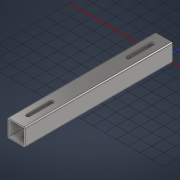
# Autodesk Inventor part: member_vertical
Saved by Autodesk Inventor 2021 (Build 250183000, 183)
## iProperties
Created: 2021-06-01
Part Number: member_vertical
Material: Steel, Galvanized
Document SubType Name: Modeling
Designer: Watchdog
Density: 7.85 g/cm^3
Appearance: Galvanized
Author: Watchdog
Autodesk Inventor part; units mm, degrees
ref_plane "YZ Plane" through (0, 0, 0) normal (1, 0, 0) x (0, 1, 0)
ref_plane "XZ Plane" through (0, 0, 0) normal (0, 1, 0) x (-1, 0, 0)
ref_plane "XY Plane" through (0, 0, 0) normal (0, 0, 1) x (1, 0, 0)
sketch "Sketch1" plane through (0, 0, 0) normal (0, 0, 1) x (1, 0, 0)
  line L0 (-15, 15) -> (15, 15)
  line L1 (15, 15) -> (15, -15)
  line L2 (15, -15) -> (-15, -15)
  line L3 (-15, -15) -> (-15, 15)
  line L4 (12.5, 12.5) -> (-12.5, 12.5)
  line L5 (-12.5, 12.5) -> (-12.5, -12.5)
  line L6 (-12.5, -12.5) -> (12.5, -12.5)
  line L7 (12.5, -12.5) -> (12.5, 12.5)
  point P0 (0, 0)
  dimension "d0" = 30
  dimension "d1" = 30
  dimension "d2" = 15
  dimension "d3" = 15
  dimension "d4" = 2.5
  constraints: 16 end point, 4 parallel, 2 perpendicular, 1 horizontal, 3 other
  measures "d0" distance of L0.start L0.end
  measures "d1" distance of L2.end L0.start
  measures "d2" distance from line of point (0, 0) L0
  measures "d3" distance from line of point (0, 0) L3
  measures "d4" distance between parallel lines of L0 L4
extrude "Extrusion1" add sketch "Sketch1" along normal blind 1000
fillet "Fillet1" radius 2 4 edges at (15, 15, 500) (-15, 15, 500) (-15, -15, 500) (15, -15, 500)
ref_plane "Work Plane1" through (0, 0, 250) normal (0, 0, -1) x (-1, 0, 0)
split "Split1" plane through (0, 0, 250) removes the side toward (0, 0, 1)
ref_plane "midPlane" through (-13, -15, 125) normal (0, 0, 1) x (1, 0, 0)
sketch "Sketch3" plane through (-13, 15, 0) normal (0, 1, 0) x (1, 0, 0)
  line L0 (13, -230) -> (13, -190) construction
  line L1 (16, -230) -> (16, -190)
  line L2 (10, -190) -> (10, -230)
  arc A0 (10, -230) -> (16, -230) centre (13, -230) ccw
  arc A1 (16, -190) -> (10, -190) centre (13, -190) ccw
  line L3 (13, -60) -> (13, -20) construction
  line L4 (16, -60) -> (16, -20)
  line L5 (10, -20) -> (10, -60)
  arc A2 (10, -60) -> (16, -60) centre (13, -60) ccw
  arc A3 (16, -20) -> (10, -20) centre (13, -20) ccw
  line L6 (28, -250) -> (28, 0) projected
  line L7 (-2, 0) -> (-2, -250) projected
  line L8 (0, -250) -> (26, -250) projected
  point P0 (13, 0)
  point P1 (13, -210)
  point P2 (13, -40)
  dimension "d28" = 6
  dimension "d29" = 6
  dimension "d30" = 30
  dimension "d31" = 15
  dimension "d32" = 15
  dimension "d33" = 40
  dimension "d34" = 40
  dimension "d35" = 20
  dimension "d36" = 20
  constraints: 16 end point, 8 point on circle, 8 tangent, 4 centre point, 2 midpoint, 2 parallel, 2 vertical
  measures "d28" diameter of A1
  measures "d29" diameter of A3
  measures "d30" distance between parallel lines of L6 L7
  measures "d31" distance between parallel lines of L7 L0
  measures "d32" distance between parallel lines of L7 L3
  measures "d33" distance of L0.end L0.start
  measures "d34" distance of L3.end L3.start
  measures "d35" distance from line of L8 L0.start
  measures "d36" distance of point (13, 0) L3.end
extrude "Extrusion2" cut sketch "Sketch3" against normal through all
equation "\"d0\" = sm_varx_squareBarDimension"
equation "\"d1\" = d0"
equation "\"d2\" = 0.5 * d1"
equation "\"d3\" = 0.5 * d0"
equation "\"d4\" = sm_varx_squareBarThickness"
equation "\"d31\" = 0.5 * d30"
equation "\"d32\" = d31"
equation "\"d34\" = d33"
equation "\"d36\" = d35"
equation "\"hoop_angle_z\" = 45deg"
equation "\"hoop_bearing_length\" = 5deg"
equation "\"hoop_cable_diam\" = 5"
equation "\"hoop_cable_pulley_diam\" = 22"
equation "\"hoop_thickness_large\" = 4"
equation "\"hoop_thickness_medium\" = 3.2"
equation "\"hoop_thickness_small\" = 2"
equation "\"hoop_width_large\" = 51"
equation "\"hoop_width_medium\" = 33.7"
equation "\"hoop_width_small\" = 25.4"
equation "\"rack_tooth_addendum\" = 5"
equation "\"rack_tooth_dedendum\" = 5"
equation "\"rack_tooth_thickness\" = 5"
equation "\"secure_arm_angle\" = 35deg"
equation "\"secure_arm_radii\" = 9"
equation "\"support_baseClamp_platformLengthBuffer\" = 35"
equation "\"support_baseClamp_platformThickness\" = 15"
equation "\"support_baseClamp_platformWidthBuffer\" = 0"
equation "\"support_baseClamp_sleeveHoleDiameter\" = 12"
equation "\"support_baseClamp_sleeveSweepTerminationAngle\" = 55deg"
equation "\"support_baseClamp_thickness\" = 8"
equation "\"support_frame_endHoleBuffer\" = 25"
equation "\"support_frame_squareBarFillet\" = 2"
equation "\"support_frame_squareBarThickness\" = 5"
equation "\"hoop_tabs_thickness\" = 6"
equation "\"hoop_tabs_hole\" = 12"
equation "\"wheelchair_deployed_width\" = 635"
equation "\"wheelchair_deployed_length\" = 1067"
equation "\"wheelchair_deployed_height\" = 914"
equation "\"sm_varx_squareBarDimension\" = 30"
equation "\"sm_varx_squareBarThickness\" = 2.5"
equation "\"sm_varx_member_tolerance\" = 0.5"
equation "\"sm_varx_pinPlate_thickness\" = 5"
equation "\"sm_varx_pinPlate_holeDiameter\" = 5"
equation "\"hoop_bushing12_radialInterference\" = 0"
equation "\"hoop_bushing23_radialInterference\" = 0"
equation "\"hoop_bushing23_od\" = -2 * hoop_thickness_medium + hoop_width_medium + hoop_bushing23_radialInterference"
body "Solid1"
